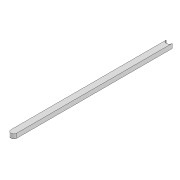
# Autodesk Inventor part: Extension_adapter
Saved by Autodesk Inventor 2022 (Build 260153000, 153)
## iProperties
Created: 2022-04-27
Part Number: Extension_adapter
Material: Generic
Document SubType Name: Modeling
Designer: dell
Density: 1 g/cm^3
Appearance: Default
Author: dell
Autodesk Inventor part; units mm, degrees
ref_plane "YZ Plane" through (0, 0, 0) normal (1, 0, 0) x (0, 1, 0)
ref_plane "XZ Plane" through (0, 0, 0) normal (0, 1, 0) x (-1, 0, 0)
ref_plane "XY Plane" through (0, 0, 0) normal (0, 0, 1) x (1, 0, 0)
sketch "Sketch1" plane through (0, 0, 0) normal (0, 1, 0) x (-1, 0, 0)
  line L0 (0, 0) -> (0, -210) construction
  line L1 (-4, 0) -> (-4, -210)
  line L2 (4, -210) -> (4, 0)
  arc A0 (4, 0) -> (-4, 0) centre (0, 0) ccw
  arc A1 (-4, -210) -> (4, -210) centre (0, -210) ccw
  circle A2 centre (0, -210) radius 4
  point P0 (0, -105)
  point P1 (4, -210)
  dimension "d0" = 210
  dimension "d1" = 8
  constraints: 8 end point, 4 point on circle, 4 tangent, 3 centre point, 1 coincident, 1 concentric, 1 midpoint, 1 parallel, 1 vertical
  measures "d0" distance of L0.start L0.end
  measures "d1" diameter of A1
extrude "Extrusion1" add sketch "Sketch1" along normal blind 6 contours A0 L2 A2 L1
body "Solid1"
